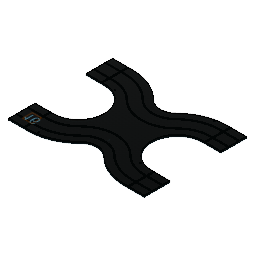
_10-16 (4-Way).ce05d46f-5f67-4321-aa04-e0567a5c2ecf (Autodesk Fusion 360 design; units mm, degrees)
Autodesk Fusion 360 part; units mm, degrees
note: some values were not read from the file. Set by a fixed rule: which sketch regions a step uses.
(part 1 of 2)
sketch "Sketch1" plane through (0, 0, 0) normal (0, 0, 1) x (1, 0, 0)
  line L0 (4241.8, -25.4) -> (3632.2, -25.4)
  line L1 (3632.2, -25.4) -> (3632.2, -838.2)
  line L2 (3632.2, -838.2) -> (4241.8, -838.2)
  line L3 (4241.8, -838.2) -> (4241.8, -25.4)
  line L4 (4241.8, -2438.4) -> (3632.2, -2438.4)
  line L5 (3632.2, -2438.4) -> (3632.2, -3251.2)
  line L6 (3632.2, -3251.2) -> (4241.8, -3251.2)
  line L7 (4241.8, -3251.2) -> (4241.8, -2438.4)
  line L8 (3632.2, -2438.4) -> (3632.2, -1638.3)
  line L9 (3632.2, -1638.3) -> (2870.2, -1638.3)
  circle A0 centre (3671.2525, -1638.3) radius 801.0525
  circle A1 centre (3632.2, -1638.3) radius 1612.9
  line L10 (0, 0) -> (609.6, 0)
  line L11 (609.6, 0) -> (609.6, -838.2)
  line L12 (609.6, -838.2) -> (0, -838.2)
  line L13 (0, -838.2) -> (0, 0)
  line L14 (0, -838.2) -> (0, -2438.4)
  line L15 (0, -2438.4) -> (609.6, -2438.4)
  line L16 (609.6, -2438.4) -> (609.6, -3276.6)
  line L17 (609.6, -3276.6) -> (0, -3276.6)
  line L18 (0, -3276.6) -> (0, -2438.4)
  line L19 (609.6, -838.2) -> (609.6, -2438.4)
  line L20 (609.6, -2438.4) -> (609.6, -1638.3)
  line L21 (609.6, -1638.3) -> (1371.6, -1638.3)
  circle A2 centre (570.5475, -1638.3) radius 801.0525
  circle A3 centre (609.6, -1638.3) radius 1638.3
  line L22 (3671.2525, -1638.3) -> (2870.2, -1638.3)
  line L23 (1371.6, -1638.3) -> (2870.2, -1638.3)
  line L24 (2120.9, -1638.3) -> (2120.9, -2635.25)
  line L25 (0, 0) -> (3390.4282, 0)
  line L26 (2065.6971, 0) -> (2065.6971, -635)
  circle A4 centre (2138.8294, -132.2917) radius 508
  circle A5 centre (2138.8294, -3144.3083) radius 508
  point P0 (2134.5605, -1039.5326)
  dimension "d8" = 609.6
  dimension "d9" = 812.8
  dimension "d12" = 812.8
  dimension "d13" = 800.1
  dimension "d14" = 762
  dimension "d15" = 609.6
  dimension "d16" = 838.2
  dimension "d17" = 1600.2
  dimension "d18" = 609.6
  dimension "d19" = 838.2
  dimension "d20" = 762
  dimension "d23" = 996.95
  dimension "d25" = 635
  dimension "d26" = 1016
  constraint horizontal L0
  constraint vertical L1
  constraint horizontal L2
  constraint vertical L3
  constraint horizontal L4
  constraint vertical L5
  constraint horizontal L6
  constraint vertical L7
  constraint perpendicular L2 L8
  constraint perpendicular L8 L9
  constraint coincident L1.end A0
  constraint coincident L9.end A0
  constraint coincident L4.end A0
  constraint coincident L5.end A1
  constraint tangent L6 A1
  constraint coincident L0.end A1
  constraint horizontal L10
  constraint vertical L11
  constraint horizontal L12
  constraint vertical L13
  constraint coincident L10.start L13.end
  constraint perpendicular L12 L14
  constraint horizontal L15
  constraint vertical L16
  constraint horizontal L17
  constraint vertical L18
  constraint midpoint L19 L20.end
  constraint perpendicular L19 L21
  constraint coincident L11.end A2
  constraint coincident L21.end A2
  constraint coincident L15.end A2
  constraint coincident L10.end A3
  constraint tangent L10 A3
  constraint coincident L16.end A3
  constraint coincident A0.centre L22.start
  constraint perpendicular L8 L22
  constraint parallel L22 L23
  constraint midpoint L23 L24.start
  constraint perpendicular L23 L24
  constraint coincident A3 P0
  constraint coincident A1 P0
  constraint perpendicular L3 L25
  constraint coincident L25 L26.start
  constraint perpendicular L25 L26
  constraint coincident L26.end A4
  constraint tangent A1 A4
  constraint tangent A3 A4
  constraint symmetric L23 A4 A5
  measures "d8" distance of L0.start L0.end
  measures "d9" distance of L0.start L2.end
  measures "d12" distance of L4.start L6.end
  measures "d13" distance of L4.end L8.end
  measures "d14" distance of L8.end L9.end
  measures "d15" distance of L10.start L10.end
  measures "d16" distance of L10.start L12.end
  measures "d17" distance of L12.end L14.end
  measures "d18" distance of L14.end L15.end
  measures "d19" distance of L14.end L17.end
  measures "d20" distance of L20.end L21.end
  measures "d23" distance of L24.start L24.end
  measures "d25" distance of L26.start L26.end
  measures "d26" diameter of A4
extrude "Extrude1" add sketch "Sketch1" along normal blind 50.8 contours L0 L3 A1 | L1 L2 L3 A0 A1 | L1 A0 A1 A3 L23 | A1 A3 A4 | L5 A0 A1 A3 L23 | A1 A3 L23 | A1 L11 A2 A3 L23 | L4 L5 L7 A0 A1 | L6 L7 A1 | A1 A3 L23 L24 | A1 L23 L24 | A1 L16 A2 A3 L23 L24 | A1 A3 A5 | L10 L13 A3 L25 | L11 L12 L13 A2 A3 | L15 L16 L18 A2 A3 | L17 L18 A3
sketch "Sketch2" plane through (0, 0, 0) normal (0, 0, -1) x (1, 0, 0)
  line L0 (2120.9, 2201.6993) -> (2120.9, 2270.7549)
  arc A0 (2134.5605, 2237.0674) -> (2120.9, 2270.7549) centre (609.6, 1638.3) ccw
  arc A1 (2134.5605, 2237.0674) -> (2120.9, 2201.6993) centre (3632.2, 1638.3) ccw
  line L1 (609.6, 3276.6) -> (0, 3276.6)
  line L2 (0, 3276.6) -> (0, 2438.4)
  line L3 (0, 2438.4) -> (531.495, 2438.4)
  arc A2 (531.495, 838.2) -> (531.495, 2438.4) centre (570.5475, 1638.3) ccw
  line L4 (531.495, 838.2) -> (0, 838.2)
  line L5 (0, 838.2) -> (0, 0)
  line L6 (0, 0) -> (609.6, 0)
  arc A3 (609.6, 0) -> (1776.8816, 488.7433) centre (609.6, 1638.3) ccw
  arc A4 (2496.523, 493.0122) -> (1776.8816, 488.7433) centre (2138.8294, 132.2917) ccw
  arc A5 (2496.523, 493.0122) -> (3632.2, 25.4) centre (3632.2, 1638.3) ccw
  line L7 (3632.2, 25.4) -> (4241.8, 25.4)
  line L8 (4241.8, 25.4) -> (4241.8, 838.2)
  line L9 (4241.8, 838.2) -> (3710.305, 838.2)
  arc A6 (3710.305, 2438.4) -> (3710.305, 838.2) centre (3671.2525, 1638.3) ccw
  line L10 (3710.305, 2438.4) -> (4241.8, 2438.4)
  line L11 (4241.8, 2438.4) -> (4241.8, 3251.2)
  line L12 (4241.8, 3251.2) -> (3632.2, 3251.2)
  arc A7 (3632.2, 3251.2) -> (2496.523, 2783.5878) centre (3632.2, 1638.3) ccw
  arc A8 (1776.8816, 2787.8567) -> (2496.523, 2783.5878) centre (2138.8294, 3144.3083) ccw
  arc A9 (1776.8816, 2787.8567) -> (609.6, 3276.6) centre (609.6, 1638.3) ccw
  line L13 (171.9803, 2701.7796) -> (461.5303, 2701.7796) construction
  line L14 (461.5303, 2701.7796) -> (461.5303, 3002.9116) construction
  line L15 (461.5303, 3002.9116) -> (171.9803, 3002.9116) construction
  line L16 (171.9803, 3002.9116) -> (171.9803, 2701.7796) construction
  dimension "d29" = 254
sketch "Sketch3" plane through (0, 0, 50.8) normal (0, 0, 1) x (-1, 0, 0)
  line L0 (-2120.9, 2270.7549) -> (-2120.9, 2201.6993)
  arc A0 (-2120.9, 2201.6993) -> (-2134.5605, 2237.0674) centre (-3632.2, 1638.3) ccw
  arc A1 (-2120.9, 2270.7549) -> (-2134.5605, 2237.0674) centre (-609.6, 1638.3) ccw
  line L1 (0, 3276.6) -> (-609.6, 3276.6)
  arc A2 (-609.6, 3276.6) -> (-1776.8816, 2787.8567) centre (-609.6, 1638.3) ccw
  arc A3 (-2496.523, 2783.5878) -> (-1776.8816, 2787.8567) centre (-2138.8294, 3144.3083) ccw
  arc A4 (-2496.523, 2783.5878) -> (-3632.2, 3251.2) centre (-3632.2, 1638.3) ccw
  line L2 (-3632.2, 3251.2) -> (-4241.8, 3251.2)
  line L3 (-4241.8, 3251.2) -> (-4241.8, 2438.4)
  line L4 (-4241.8, 2438.4) -> (-3710.305, 2438.4)
  arc A5 (-3710.305, 838.2) -> (-3710.305, 2438.4) centre (-3671.2525, 1638.3) ccw
  line L5 (-3710.305, 838.2) -> (-4241.8, 838.2)
  line L6 (-4241.8, 838.2) -> (-4241.8, 25.4)
  line L7 (-4241.8, 25.4) -> (-3632.2, 25.4)
  arc A6 (-3632.2, 25.4) -> (-2496.523, 493.0122) centre (-3632.2, 1638.3) ccw
  arc A7 (-1776.8816, 488.7433) -> (-2496.523, 493.0122) centre (-2138.8294, 132.2917) ccw
  arc A8 (-1776.8816, 488.7433) -> (-609.6, 0) centre (-609.6, 1638.3) ccw
  line L8 (-609.6, 0) -> (0, 0)
  line L9 (0, 0) -> (0, 838.2)
  line L10 (0, 838.2) -> (-531.495, 838.2)
  arc A9 (-531.495, 2438.4) -> (-531.495, 838.2) centre (-570.5475, 1638.3) ccw
  line L11 (-531.495, 2438.4) -> (0, 2438.4)
  line L12 (0, 2438.4) -> (0, 3276.6)
extrude "Extrude2" add sketch "Sketch3" against normal blind 50.8 contours L0 A0 A1
sketch "Sketch4" plane through (0, 0, 50.8) normal (0, 0, 1) x (-1, 0, 0)
  line L0 (0, 3276.6) -> (-609.6, 3276.6)
  arc A0 (-609.6, 3276.6) -> (-1776.8816, 2787.8567) centre (-609.6, 1638.3) ccw
  arc A1 (-2496.523, 2783.5878) -> (-1776.8816, 2787.8567) centre (-2138.8294, 3144.3083) ccw
  arc A2 (-2496.523, 2783.5878) -> (-3632.2, 3251.2) centre (-3632.2, 1638.3) ccw
  line L1 (-3632.2, 3251.2) -> (-4241.8, 3251.2)
  line L2 (-4241.8, 3251.2) -> (-4241.8, 2438.4)
  line L3 (-4241.8, 2438.4) -> (-3710.305, 2438.4)
  arc A3 (-3710.305, 838.2) -> (-3710.305, 2438.4) centre (-3671.2525, 1638.3) ccw
  line L4 (-3710.305, 838.2) -> (-4241.8, 838.2)
  line L5 (-4241.8, 838.2) -> (-4241.8, 25.4)
  line L6 (-4241.8, 25.4) -> (-3632.2, 25.4)
  arc A4 (-3632.2, 25.4) -> (-2496.523, 493.0122) centre (-3632.2, 1638.3) ccw
  arc A5 (-1776.8816, 488.7433) -> (-2496.523, 493.0122) centre (-2138.8294, 132.2917) ccw
  arc A6 (-1776.8816, 488.7433) -> (-609.6, 0) centre (-609.6, 1638.3) ccw
  line L7 (-609.6, 0) -> (0, 0)
  line L8 (0, 0) -> (0, 838.2)
  line L9 (0, 838.2) -> (-531.495, 838.2)
  arc A7 (-531.495, 2438.4) -> (-531.495, 838.2) centre (-570.5475, 1638.3) ccw
  line L10 (-531.495, 2438.4) -> (0, 2438.4)
  line L11 (0, 2438.4) -> (0, 3276.6)
  line L12 (-4241.8, 838.2) -> (-2590.8, 838.2)
  line L13 (-2590.8, 838.2) -> (-2590.8, 508)
  circle A8 centre (-2590.8, 508) radius 16
  dimension "d35" = 1651
  dimension "d37" = 330.2
  dimension "d38" = 32
  constraint coincident L4.end L5.start
  constraint perpendicular L5 L12
  constraint perpendicular L12 L13
  constraint coincident L13.end A8.centre
  measures "d35" distance of L4.end L12.end
  measures "d37" distance of L12.end L13.end
  measures "d38" diameter of A8
extrude "Extrude3" add sketch "Sketch4" along normal blind 0.0254 contours A8
sketch "Sketch5" plane through (0, 0, 50.8) normal (0, 0, 1) x (-1, 0, 0)
  circle A0 centre (-2590.8, 508) radius 16
  line L0 (0, 3276.6) -> (-609.6, 3276.6)
  arc A1 (-609.6, 3276.6) -> (-1776.8816, 2787.8567) centre (-609.6, 1638.3) ccw
  arc A2 (-2496.523, 2783.5878) -> (-1776.8816, 2787.8567) centre (-2138.8294, 3144.3083) ccw
  arc A3 (-2496.523, 2783.5878) -> (-3632.2, 3251.2) centre (-3632.2, 1638.3) ccw
  line L1 (-3632.2, 3251.2) -> (-4241.8, 3251.2)
  line L2 (-4241.8, 3251.2) -> (-4241.8, 2438.4)
  line L3 (-4241.8, 2438.4) -> (-3710.305, 2438.4)
  line L4 (-3710.305, 838.2) -> (-4241.8, 838.2)
  line L5 (-4241.8, 838.2) -> (-4241.8, 25.4)
  line L6 (-4241.8, 25.4) -> (-3632.2, 25.4)
  arc A4 (-1776.8816, 488.7433) -> (-2496.523, 493.0122) centre (-2138.8294, 132.2917) ccw
  arc A5 (-1776.8816, 488.7433) -> (-609.6, 0) centre (-609.6, 1638.3) ccw
  line L7 (-609.6, 0) -> (0, 0)
  line L8 (0, 0) -> (0, 838.2)
  line L9 (0, 838.2) -> (-531.495, 838.2)
  arc A6 (-531.495, 2438.4) -> (-531.495, 838.2) centre (-570.5475, 1638.3) ccw
  line L10 (-531.495, 2438.4) -> (0, 2438.4)
  line L11 (0, 2438.4) -> (0, 3276.6)
  line L12 (-3008.1535, 617.6738) -> (-2791.2306, 262.1613)
  line L13 (-3008.1535, 617.6738) -> (-2791.2306, 262.1613)
  line L14 (-2791.2306, 262.1613) -> (-2802.0718, 255.5463)
  line L15 (-2802.0718, 255.5463) -> (-3018.9947, 611.0588)
  line L16 (-3018.9947, 611.0588) -> (-3008.1535, 617.6738)
  point P0 (-3225.0764, 973.1864)
  point P1 (-2791.2306, 262.1613)
  point P2 (-3008.1535, 617.6738)
  dimension "d45" = 12.7
  constraint coincident P2 L12.start
  constraint coincident P1 L12.end
  constraint perpendicular L13 L14
  constraint parallel L13 L15
  constraint parallel L14 L16
  constraint parallel L12 L13
  measures "d45" distance of P2 L15.end
extrude "Extrude4" add sketch "Sketch5" along normal blind 0.0254 contours L12 L13 L14 L15 L16
extrude "Extrude5" cut sketch "Sketch5" along normal blind 0.0254 contours L12 L13 L14 L15 L16
extrude "Extrude6" add sketch "Sketch5" along normal blind 0.0254 contours L12 L13 L14 L15 L16
sketch "Sketch6" plane through (0, 0, 50.8) normal (0, 0, 1) x (-1, 0, 0)
  line L0 (-3018.9947, 611.0588) -> (-3008.1535, 617.6738)
  line L1 (-3008.1535, 617.6738) -> (-2791.2306, 262.1613)
  line L2 (-2791.2306, 262.1613) -> (-2802.0718, 255.5463)
  line L3 (-2802.0718, 255.5463) -> (-3018.9947, 611.0588)
  circle A0 centre (-2590.8, 508) radius 16
  line L4 (0, 3276.6) -> (-609.6, 3276.6)
  arc A1 (-609.6, 3276.6) -> (-1776.8816, 2787.8567) centre (-609.6, 1638.3) ccw
  arc A2 (-2496.523, 2783.5878) -> (-1776.8816, 2787.8567) centre (-2138.8294, 3144.3083) ccw
  arc A3 (-2496.523, 2783.5878) -> (-3632.2, 3251.2) centre (-3632.2, 1638.3) ccw
  line L5 (-3632.2, 3251.2) -> (-4241.8, 3251.2)
  line L6 (-4241.8, 3251.2) -> (-4241.8, 2438.4)
  line L7 (-4241.8, 2438.4) -> (-3710.305, 2438.4)
  arc A4 (-3710.305, 838.2) -> (-3710.305, 2438.4) centre (-3671.2525, 1638.3) ccw
  line L8 (-3710.305, 838.2) -> (-4241.8, 838.2)
  line L9 (-4241.8, 838.2) -> (-4241.8, 25.4)
  line L10 (-4241.8, 25.4) -> (-3632.2, 25.4)
  arc A5 (-3632.2, 25.4) -> (-2496.523, 493.0122) centre (-3632.2, 1638.3) ccw
  arc A6 (-1776.8816, 488.7433) -> (-2496.523, 493.0122) centre (-2138.8294, 132.2917) ccw
  arc A7 (-1776.8816, 488.7433) -> (-609.6, 0) centre (-609.6, 1638.3) ccw
  line L11 (-609.6, 0) -> (0, 0)
  line L12 (0, 0) -> (0, 838.2)
  line L13 (0, 838.2) -> (-531.495, 838.2)
  arc A8 (-531.495, 2438.4) -> (-531.495, 838.2) centre (-570.5475, 1638.3) ccw
  line L14 (-531.495, 2438.4) -> (0, 2438.4)
  line L15 (0, 2438.4) -> (0, 3276.6)
extrude "Extrude7" cut 1 faces at (2867.152, -378.4604, 50.8254) along direction (0, 0, -1) blind 0.0254
extrude "Extrude8" cut 1 faces at (2591.9868, -520.4548, 50.8254) along direction (0, 0, -1) blind 0.0254
sketch "Sketch7" plane through (0, 0, 50.8) normal (0, 0, 1) x (-1, 0, 0)
  line L0 (0, 3276.6) -> (-609.6, 3276.6)
  arc A0 (-609.6, 3276.6) -> (-1776.8816, 2787.8567) centre (-609.6, 1638.3) ccw
  arc A1 (-2496.523, 2783.5878) -> (-1776.8816, 2787.8567) centre (-2138.8294, 3144.3083) ccw
  arc A2 (-2496.523, 2783.5878) -> (-3632.2, 3251.2) centre (-3632.2, 1638.3) ccw
  line L1 (-3632.2, 3251.2) -> (-4241.8, 3251.2)
  line L2 (-4241.8, 3251.2) -> (-4241.8, 2438.4)
  line L3 (-4241.8, 2438.4) -> (-3710.305, 2438.4)
  arc A3 (-3710.305, 838.2) -> (-3710.305, 2438.4) centre (-3671.2525, 1638.3) ccw
  line L4 (-3710.305, 838.2) -> (-4241.8, 838.2)
  line L5 (-4241.8, 838.2) -> (-4241.8, 25.4)
  line L6 (-4241.8, 25.4) -> (-3632.2, 25.4)
  arc A4 (-3632.2, 25.4) -> (-2496.523, 493.0122) centre (-3632.2, 1638.3) ccw
  arc A5 (-1776.8816, 488.7433) -> (-2496.523, 493.0122) centre (-2138.8294, 132.2917) ccw
  arc A6 (-1776.8816, 488.7433) -> (-609.6, 0) centre (-609.6, 1638.3) ccw
  line L7 (-609.6, 0) -> (0, 0)
  line L8 (0, 0) -> (0, 838.2)
  line L9 (0, 838.2) -> (-531.495, 838.2)
  arc A7 (-531.495, 2438.4) -> (-531.495, 838.2) centre (-570.5475, 1638.3) ccw
  line L10 (-531.495, 2438.4) -> (0, 2438.4)
  line L11 (0, 2438.4) -> (0, 3276.6)
  line L12 (-3759.2, 741.3544) -> (-3759.2, 838.2)
  line L13 (-3759.2, 741.3544) -> (-3759.2, 25.4)
  line L14 (-3759.2, 838.2) -> (-3730.625, 838.2)
  line L15 (-3730.625, 838.2) -> (-3730.625, 25.4)
  line L16 (-3730.625, 25.4) -> (-3759.2, 25.4)
  line L17 (-3759.2, 838.2) -> (-3730.625, 838.2)
  line L18 (-3759.2, 838.2) -> (-3730.625, 838.2)
  line L19 (-3730.625, 838.2) -> (-3730.625, 25.4)
  line L20 (-3730.625, 25.4) -> (-3759.2, 25.4)
  line L21 (-3759.2, 25.4) -> (-3759.2, 838.2)
  constraint coincident L4 L12.end
  constraint perpendicular L4 L12
  constraint coincident L6 L13.end
  constraint perpendicular L6 L13
  constraint coincident L6 L15.end
  constraint perpendicular L6 L15
  constraint perpendicular L15 L17
  constraint horizontal L18
  constraint vertical L19
  constraint horizontal L20
  constraint vertical L21
extrude "Extrude9" add sketch "Sketch7" along normal blind 0.0254 contours L4 L6 L12 L13 L14 L15 L16 L17 L18 L19 L20 L21
sketch "Sketch8" plane through (0, 0, 50.8) normal (0, 0, 1) x (-1, 0, 0)
  line L0 (-3730.625, 838.2) -> (-3730.625, 25.4)
  line L1 (-3730.625, 25.4) -> (-3632.2, 25.4)
  arc A0 (-3632.2, 25.4) -> (-2496.523, 493.0122) centre (-3632.2, 1638.3) ccw
  arc A1 (-1776.8816, 488.7433) -> (-2496.523, 493.0122) centre (-2138.8294, 132.2917) ccw
  arc A2 (-1776.8816, 488.7433) -> (-609.6, 0) centre (-609.6, 1638.3) ccw
  line L2 (-609.6, 0) -> (0, 0)
  line L3 (0, 0) -> (0, 838.2)
  line L4 (0, 838.2) -> (-531.495, 838.2)
  arc A3 (-531.495, 2438.4) -> (-531.495, 838.2) centre (-570.5475, 1638.3) ccw
  line L5 (-531.495, 2438.4) -> (0, 2438.4)
  line L6 (0, 2438.4) -> (0, 3276.6)
  line L7 (0, 3276.6) -> (-609.6, 3276.6)
  arc A4 (-609.6, 3276.6) -> (-1776.8816, 2787.8567) centre (-609.6, 1638.3) ccw
  arc A5 (-2496.523, 2783.5878) -> (-1776.8816, 2787.8567) centre (-2138.8294, 3144.3083) ccw
  arc A6 (-2496.523, 2783.5878) -> (-3632.2, 3251.2) centre (-3632.2, 1638.3) ccw
  line L8 (-3632.2, 3251.2) -> (-4241.8, 3251.2)
  line L9 (-4241.8, 3251.2) -> (-4241.8, 2438.4)
  line L10 (-4241.8, 2438.4) -> (-3710.305, 2438.4)
  arc A7 (-3710.305, 838.2) -> (-3710.305, 2438.4) centre (-3671.2525, 1638.3) ccw
  line L11 (-3710.305, 838.2) -> (-3730.625, 838.2)
sketch "Sketch9" plane through (0, 0, 50.8) normal (0, 0, 1) x (-1, 0, 0)
  line L0 (0, 431.8) -> (-482.6, 431.8)
  line L1 (-482.6, 431.8) -> (-482.6, 838.2)
  line L2 (-482.6, 838.2) -> (-511.175, 838.2)
  line L3 (-511.175, 838.2) -> (-511.175, -0.0124)
  line L4 (-511.175, -0.0124) -> (-482.6, -0.0124)
  line L5 (-482.6, -0.0124) -> (-482.6, 838.2)
  line L6 (0, 2870.2) -> (-482.6, 2870.2)
  line L7 (-4241.7999, 2844.8) -> (-3759.1999, 2844.8)
  line L8 (-3759.1999, 2844.8) -> (-3730.6249, 2844.8)
  line L9 (-3730.6249, 2844.8) -> (-3730.6249, 2438.5075)
  line L10 (-3730.6249, 2438.5075) -> (-3759.1999, 2438.5075)
  line L11 (-3759.1999, 2438.5075) -> (-3759.1999, 2844.8)
  line L12 (-3730.6249, 2844.8) -> (-3759.1999, 2844.8)
  line L13 (-3759.1999, 2844.8) -> (-3759.1999, 3251.2)
  line L14 (-3759.1999, 3251.2) -> (-3730.6249, 3251.2)
  line L15 (-3730.6249, 3251.2) -> (-3730.6249, 2844.8)
  line L16 (-482.6, 2870.2) -> (-511.175, 2870.2)
  line L17 (-511.175, 2870.2) -> (-511.175, 2438.6051)
  line L18 (-511.175, 2438.6051) -> (-482.6, 2438.6051)
  line L19 (-482.6, 2438.6051) -> (-482.6, 2870.2)
  line L20 (-482.6, 2870.2) -> (-511.175, 2870.2)
  line L21 (-511.175, 2870.2) -> (-511.175, 3276.173)
  line L22 (-511.175, 3276.173) -> (-482.6, 3276.173)
  line L23 (-482.6, 3276.173) -> (-482.6, 2870.2)
  line L24 (-3730.625, 838.2) -> (-3730.625, 25.4)
  line L25 (-3730.625, 25.4) -> (-3632.2, 25.4)
  arc A0 (-3632.2, 25.4) -> (-2496.523, 493.0122) centre (-3632.2, 1638.3) ccw
  arc A1 (-1776.8816, 488.7433) -> (-2496.523, 493.0122) centre (-2138.8294, 132.2917) ccw
  arc A2 (-1776.8816, 488.7433) -> (-609.6, 0) centre (-609.6, 1638.3) ccw
  line L26 (-609.6, 0) -> (0, 0)
  line L27 (0, 0) -> (0, 838.2)
  line L28 (0, 838.2) -> (-531.495, 838.2)
  arc A3 (-531.495, 2438.4) -> (-531.495, 838.2) centre (-570.5475, 1638.3) ccw
  line L29 (-531.495, 2438.4) -> (0, 2438.4)
  line L30 (0, 2438.4) -> (0, 3276.6)
  line L31 (0, 3276.6) -> (-609.6, 3276.6)
  arc A4 (-609.6, 3276.6) -> (-1776.8816, 2787.8567) centre (-609.6, 1638.3) ccw
  arc A5 (-2496.523, 2783.5878) -> (-1776.8816, 2787.8567) centre (-2138.8294, 3144.3083) ccw
  arc A6 (-2496.523, 2783.5878) -> (-3632.2, 3251.2) centre (-3632.2, 1638.3) ccw
  line L32 (-3632.2, 3251.2) -> (-4241.8, 3251.2)
  line L33 (-4241.8, 3251.2) -> (-4241.8, 2438.4)
  line L34 (-4241.8, 2438.4) -> (-3710.305, 2438.4)
  arc A7 (-3710.305, 838.2) -> (-3710.305, 2438.4) centre (-3671.2525, 1638.3) ccw
  line L35 (-3710.305, 838.2) -> (-3730.625, 838.2)
  line L36 (-4241.8, 25.4) -> (-3632.2, 25.4)
  line L37 (-3710.305, 838.2) -> (-4241.8, 838.2)
  line L38 (-4241.8, 838.2) -> (-4241.8, 25.4)
  line L39 (-63.5, 774.7) -> (-529.9758, 774.7)
  arc A8 (-529.9758, 2501.9) -> (-529.9758, 774.7) centre (-570.5475, 1638.3) ccw
  line L40 (-529.9758, 2501.9) -> (-63.5, 2501.9)
  line L41 (-63.5, 2501.9) -> (-63.5, 3213.1)
  line L42 (-63.5, 3213.1) -> (-609.6, 3213.1)
  arc A9 (-609.6, 3213.1) -> (-1731.6381, 2743.3002) centre (-609.6, 1638.3) ccw
  arc A10 (-2541.2347, 2738.4977) -> (-1731.6381, 2743.3002) centre (-2138.8294, 3144.3083) ccw
  arc A11 (-2541.2347, 2738.4977) -> (-3632.2, 3187.7) centre (-3632.2, 1638.3) ccw
  line L43 (-3632.2, 3187.7) -> (-4178.3, 3187.7)
  line L44 (-4178.3, 3187.7) -> (-4178.3, 2501.9)
  line L45 (-4178.3, 2501.9) -> (-3711.8242, 2501.9)
  arc A12 (-3667.125, 773.7574) -> (-3711.8242, 2501.9) centre (-3671.2525, 1638.3) ccw
  line L46 (-3667.125, 773.7574) -> (-3667.125, 88.9)
  line L47 (-3667.125, 88.9) -> (-3632.2, 88.9)
  arc A13 (-3632.2, 88.9) -> (-2541.2347, 538.1023) centre (-3632.2, 1638.3) ccw
  arc A14 (-1731.6381, 533.2998) -> (-2541.2347, 538.1023) centre (-2138.8294, 132.2917) ccw
  arc A15 (-1731.6381, 533.2998) -> (-609.6, 63.5) centre (-609.6, 1638.3) ccw
  line L48 (-609.6, 63.5) -> (-63.5, 63.5)
  line L49 (-63.5, 63.5) -> (-63.5, 774.7)
  circle A16 centre (-3302, 2420.0312) radius 16
  circle A17 centre (-863.6, 3192.4811) radius 16
  circle A18 centre (-914.4, 845.0683) radius 16
  circle A19 centre (-3314.7, 121.7796) radius 16
  dimension "d60" = 482.6
  dimension "d61" = 28.575
  dimension "d62" = 482.6
  dimension "d63" = 482.6
  dimension "d64" = 28.575
  dimension "d65" = 28.575
  dimension "d66" = 63.5
  dimension "d70" = 32
  dimension "d72" = 32
  dimension "d74" = 32
  dimension "d76" = 32
  constraint horizontal L0
  constraint perpendicular L0 L1
  constraint horizontal L2
  constraint vertical L3
  constraint horizontal L4
  constraint vertical L5
  constraint horizontal L6
  constraint horizontal L7
  constraint horizontal L8
  constraint vertical L9
  constraint horizontal L10
  constraint vertical L11
  constraint horizontal L12
  constraint vertical L13
  constraint horizontal L14
  constraint vertical L15
  constraint horizontal L16
  constraint vertical L17
  constraint horizontal L18
  constraint vertical L19
  constraint horizontal L20
  constraint vertical L21
  constraint horizontal L22
  constraint vertical L23
  measures "d60" distance of L0.start L0.end
  measures "d61" distance of L1.end L2.end
  measures "d62" distance of L6.start L6.end
  measures "d63" distance of L7.start L7.end
  measures "d64" distance of L7.end L8.end
  measures "d65" distance of L6.end L16.end
  measures "d70" diameter of A16
  measures "d72" diameter of A17
  measures "d74" diameter of A18
  measures "d76" diameter of A19
extrude "Extrude10" add sketch "Sketch9" along normal blind 0.0254 contours L1 L3 L5 L39 L48 | L3 L5 L26 L48 | L1 L2 L3 L5 L28 L39 | L17 L18 L19 L40 | L16 L17 L19 L20 L40 | L16 L20 L21 L23 L42 | L21 L22 L23 L42 | L13 L14 L15 L32 L43 | L8 L12 L13 L15 L43 | L8 L9 L11 L12 L45 | L9 L10 L11 L45
extrude "Extrude11" add sketch "Sketch9" along normal blind 0.0254 contours A8 A18 | A8 A18 | A13 A19 | A13 A19 | A9 A17 | A9 A17 | A12 A16 | A12 A16
sketch "Sketch10" plane through (0, 0, 50.8) normal (0, 0, 1) x (-1, 0, 0)
  circle A0 centre (-3314.7, 121.7796) radius 16
  circle A1 centre (-3302, 2420.0312) radius 16
  circle A2 centre (-914.4, 845.0683) radius 16
  circle A3 centre (-863.6, 3192.4811) radius 16
  line L0 (-482.6, 838.2) -> (-482.6, 0)
  line L1 (-482.6, 0) -> (0, 0)
  line L2 (0, 0) -> (0, 838.2)
  line L3 (0, 838.2) -> (-531.495, 838.2)
  arc A4 (-531.495, 2438.4) -> (-531.495, 838.2) centre (-570.5475, 1638.3) ccw
  line L4 (-531.495, 2438.4) -> (0, 2438.4)
  line L5 (0, 2438.4) -> (0, 3276.6)
  line L6 (0, 3276.6) -> (-609.6, 3276.6)
  arc A5 (-609.6, 3276.6) -> (-1776.8816, 2787.8567) centre (-609.6, 1638.3) ccw
  arc A6 (-2496.523, 2783.5878) -> (-1776.8816, 2787.8567) centre (-2138.8294, 3144.3083) ccw
  arc A7 (-2496.523, 2783.5878) -> (-3632.2, 3251.2) centre (-3632.2, 1638.3) ccw
  line L7 (-3632.2, 3251.2) -> (-4241.8, 3251.2)
  line L8 (-4241.8, 3251.2) -> (-4241.8, 2438.4)
  line L9 (-4241.8, 2438.4) -> (-3710.305, 2438.4)
  arc A8 (-3710.305, 838.2) -> (-3710.305, 2438.4) centre (-3671.2525, 1638.3) ccw
  line L10 (-3710.305, 838.2) -> (-3730.625, 838.2)
  line L11 (-3730.625, 838.2) -> (-3730.625, 25.4)
  line L12 (-3730.625, 25.4) -> (-3632.2, 25.4)
  arc A9 (-3632.2, 25.4) -> (-2496.523, 493.0122) centre (-3632.2, 1638.3) ccw
  arc A10 (-1776.8816, 488.7433) -> (-2496.523, 493.0122) centre (-2138.8294, 132.2917) ccw
  arc A11 (-1776.8816, 488.7433) -> (-609.6, 0) centre (-609.6, 1638.3) ccw
  line L13 (-609.6, 0) -> (-511.175, 0)
  line L14 (-511.175, 0) -> (-511.175, 838.2)
  line L15 (-511.175, 838.2) -> (-482.6, 838.2)
  line L16 (-511.175, 3276.173) -> (-482.6, 3276.173)
  line L17 (-482.6, 3276.173) -> (-482.6, 2438.6051)
  line L18 (-482.6, 2438.6051) -> (-511.175, 2438.6051)
  line L19 (-511.175, 2438.6051) -> (-511.175, 3276.173)
  line L20 (-3730.6249, 3251.2) -> (-3730.6249, 2438.5075)
  line L21 (-3730.6249, 2438.5075) -> (-3759.1999, 2438.5075)
  line L22 (-3759.1999, 2438.5075) -> (-3759.1999, 3251.2)
  line L23 (-3759.1999, 3251.2) -> (-3730.6249, 3251.2)
  arc A12 (-1611.7429, 651.3744) -> (-609.6, 231.775) centre (-609.6, 1638.3) ccw
  line L24 (-609.6, 231.775) -> (-511.175, 231.775)
  arc A13 (-1598.1699, 664.7414) -> (-609.6, 250.825) centre (-609.6, 1638.3) ccw
  line L25 (-609.6, 250.825) -> (-511.175, 250.825)
  arc A14 (-1598.1699, 664.7414) -> (-2673.1342, 671.118) centre (-2138.8294, 132.2917) ccw
  arc A15 (-1611.7429, 651.3744) -> (-2659.7206, 657.591) centre (-2138.8294, 132.2917) ccw
  arc A16 (-3632.2, 257.175) -> (-2659.7206, 657.591) centre (-3632.2, 1638.3) ccw
  line L26 (-3730.625, 257.175) -> (-3632.2, 257.175)
  line L27 (-3730.625, 276.225) -> (-3632.2, 276.225)
  arc A17 (-3632.2, 276.225) -> (-2673.1342, 671.118) centre (-3632.2, 1638.3) ccw
  dimension "d79" = -231.775
  dimension "d80" = -250.825
  dimension "d81" = 250.825
  dimension "d82" = 231.775
  dimension "d85" = -250.825
extrude "Extrude12" add sketch "Sketch10" along normal blind 0.0279 contours L11 L14 A12 L24 A13 L25 A14 A15 A16 L26 L27 A17
sketch "Sketch11" plane through (0, 0, 0) normal (0, 0, -1) x (1, 0, 0)
sketch "Sketch12" plane through (0, 0, 50.8) normal (0, 0, 1) x (-1, 0, 0)
  line L0 (-609.6, 250.825) -> (-511.175, 250.825)
  line L1 (-511.175, 250.825) -> (-511.175, 838.2)
  line L2 (-511.175, 838.2) -> (-482.6, 838.2)
  line L3 (-482.6, 838.2) -> (-482.6, 0)
  line L4 (-482.6, 0) -> (0, 0)
  line L5 (0, 0) -> (0, 838.2)
  line L6 (0, 838.2) -> (-531.495, 838.2)
  arc A0 (-531.495, 2438.4) -> (-531.495, 838.2) centre (-570.5475, 1638.3) ccw
  line L7 (-531.495, 2438.4) -> (0, 2438.4)
  line L8 (0, 2438.4) -> (0, 3276.6)
  line L9 (0, 3276.6) -> (-609.6, 3276.6)
  arc A1 (-609.6, 3276.6) -> (-1776.8816, 2787.8567) centre (-609.6, 1638.3) ccw
  arc A2 (-2496.523, 2783.5878) -> (-1776.8816, 2787.8567) centre (-2138.8294, 3144.3083) ccw
  arc A3 (-2496.523, 2783.5878) -> (-3632.2, 3251.2) centre (-3632.2, 1638.3) ccw
  line L10 (-3632.2, 3251.2) -> (-4241.8, 3251.2)
  line L11 (-4241.8, 3251.2) -> (-4241.8, 2438.4)
  line L12 (-4241.8, 2438.4) -> (-3710.305, 2438.4)
  arc A4 (-3710.305, 838.2) -> (-3710.305, 2438.4) centre (-3671.2525, 1638.3) ccw
  line L13 (-3710.305, 838.2) -> (-3730.625, 838.2)
  line L14 (-3730.625, 838.2) -> (-3730.625, 276.225)
  line L15 (-3730.625, 276.225) -> (-3632.2, 276.225)
  arc A5 (-3632.2, 276.225) -> (-2673.1342, 671.118) centre (-3632.2, 1638.3) ccw
  arc A6 (-1598.1699, 664.7414) -> (-2673.1342, 671.118) centre (-2138.8294, 132.2917) ccw
  arc A7 (-1598.1699, 664.7414) -> (-609.6, 250.825) centre (-609.6, 1638.3) ccw
  circle A8 centre (-3302, 2420.0312) radius 16
  circle A9 centre (-914.4, 845.0683) radius 16
  circle A10 centre (-863.6, 3192.4811) radius 16
  line L16 (-511.175, 3276.173) -> (-482.6, 3276.173)
  line L17 (-482.6, 3276.173) -> (-482.6, 2438.6051)
  line L18 (-482.6, 2438.6051) -> (-511.175, 2438.6051)
  line L19 (-511.175, 2438.6051) -> (-511.175, 3276.173)
  line L20 (-3730.6249, 3251.2) -> (-3730.6249, 2438.5075)
  line L21 (-3730.6249, 2438.5075) -> (-3759.1999, 2438.5075)
  line L22 (-3759.1999, 2438.5075) -> (-3759.1999, 3251.2)
  line L23 (-3759.1999, 3251.2) -> (-3730.6249, 3251.2)
  line L24 (-482.6, 250.825) -> (0, 250.825)
  line L25 (-482.6, 231.775) -> (0, 231.775)
  dimension "d89" = -231.775
extrude "Extrude13" add sketch "Sketch12" along normal blind 0.0279 contours L3 L5 L24 L25
sketch "Sketch13" plane through (0, 0, 50.8) normal (0, 0, 1) x (-1, 0, 0)
  line L0 (-482.6, 250.825) -> (0, 250.825)
  line L1 (0, 250.825) -> (0, 838.2)
  line L2 (0, 838.2) -> (-531.495, 838.2)
  arc A0 (-531.495, 2438.4) -> (-531.495, 838.2) centre (-570.5475, 1638.3) ccw
  line L3 (-531.495, 2438.4) -> (0, 2438.4)
  line L4 (0, 2438.4) -> (0, 3276.6)
  line L5 (0, 3276.6) -> (-609.6, 3276.6)
  arc A1 (-609.6, 3276.6) -> (-1776.8816, 2787.8567) centre (-609.6, 1638.3) ccw
  arc A2 (-2496.523, 2783.5878) -> (-1776.8816, 2787.8567) centre (-2138.8294, 3144.3083) ccw
  arc A3 (-2496.523, 2783.5878) -> (-3632.2, 3251.2) centre (-3632.2, 1638.3) ccw
  line L6 (-3632.2, 3251.2) -> (-4241.8, 3251.2)
  line L7 (-4241.8, 3251.2) -> (-4241.8, 2438.4)
  line L8 (-4241.8, 2438.4) -> (-3710.305, 2438.4)
  arc A4 (-3710.305, 838.2) -> (-3710.305, 2438.4) centre (-3671.2525, 1638.3) ccw
  line L9 (-3710.305, 838.2) -> (-3730.625, 838.2)
  line L10 (-3730.625, 838.2) -> (-3730.625, 276.225)
  line L11 (-3730.625, 276.225) -> (-3632.2, 276.225)
  arc A5 (-3632.2, 276.225) -> (-2673.1342, 671.118) centre (-3632.2, 1638.3) ccw
  arc A6 (-1598.1699, 664.7414) -> (-2673.1342, 671.118) centre (-2138.8294, 132.2917) ccw
  arc A7 (-1598.1699, 664.7414) -> (-609.6, 250.825) centre (-609.6, 1638.3) ccw
  line L12 (-609.6, 250.825) -> (-511.175, 250.825)
  line L13 (-511.175, 250.825) -> (-511.175, 838.2)
  line L14 (-511.175, 838.2) -> (-482.6, 838.2)
  line L15 (-482.6, 838.2) -> (-482.6, 250.825)
  circle A8 centre (-3302, 2420.0312) radius 16
  circle A9 centre (-914.4, 845.0683) radius 16
  circle A10 centre (-863.6, 3192.4811) radius 16
  line L16 (-511.175, 3276.173) -> (-482.6, 3276.173)
  line L17 (-482.6, 3276.173) -> (-482.6, 2438.6051)
  line L18 (-482.6, 2438.6051) -> (-511.175, 2438.6051)
  line L19 (-511.175, 2438.6051) -> (-511.175, 3276.173)
  line L20 (-3730.6249, 3251.2) -> (-3730.6249, 2438.5075)
  line L21 (-3730.6249, 2438.5075) -> (-3759.1999, 2438.5075)
  line L22 (-3759.1999, 2438.5075) -> (-3759.1999, 3251.2)
  line L23 (-3759.1999, 3251.2) -> (-3730.6249, 3251.2)
  line L24 (0, 587.375) -> (-531.495, 587.375)
  line L25 (0, 606.425) -> (-531.495, 606.425)
  dimension "d92" = -250.825
  dimension "d93" = -231.775
extrude "Extrude14" add sketch "Sketch13" along normal blind 0.0279 contours L1 L15 L24 L25
sketch "Sketch14" plane through (0, 0, 50.8) normal (0, 0, 1) x (-1, 0, 0)
  line L0 (-482.6, 606.425) -> (0, 606.425)
  line L1 (0, 606.425) -> (0, 838.2)
  line L2 (0, 838.2) -> (-531.495, 838.2)
  arc A0 (-531.495, 2438.4) -> (-531.495, 838.2) centre (-570.5475, 1638.3) ccw
  line L3 (-531.495, 2438.4) -> (0, 2438.4)
  line L4 (0, 2438.4) -> (0, 3276.6)
  line L5 (0, 3276.6) -> (-609.6, 3276.6)
  arc A1 (-609.6, 3276.6) -> (-1776.8816, 2787.8567) centre (-609.6, 1638.3) ccw
  arc A2 (-2496.523, 2783.5878) -> (-1776.8816, 2787.8567) centre (-2138.8294, 3144.3083) ccw
  arc A3 (-2496.523, 2783.5878) -> (-3632.2, 3251.2) centre (-3632.2, 1638.3) ccw
  line L6 (-3632.2, 3251.2) -> (-4241.8, 3251.2)
  line L7 (-4241.8, 3251.2) -> (-4241.8, 2438.4)
  line L8 (-4241.8, 2438.4) -> (-3710.305, 2438.4)
  arc A4 (-3710.305, 838.2) -> (-3710.305, 2438.4) centre (-3671.2525, 1638.3) ccw
  line L9 (-3710.305, 838.2) -> (-3730.625, 838.2)
  line L10 (-3730.625, 838.2) -> (-3730.625, 276.225)
  line L11 (-3730.625, 276.225) -> (-3632.2, 276.225)
  arc A5 (-3632.2, 276.225) -> (-2673.1342, 671.118) centre (-3632.2, 1638.3) ccw
  arc A6 (-1598.1699, 664.7414) -> (-2673.1342, 671.118) centre (-2138.8294, 132.2917) ccw
  arc A7 (-1598.1699, 664.7414) -> (-609.6, 250.825) centre (-609.6, 1638.3) ccw
  line L12 (-609.6, 250.825) -> (-511.175, 250.825)
  line L13 (-511.175, 250.825) -> (-511.175, 838.2)
  line L14 (-511.175, 838.2) -> (-482.6, 838.2)
  line L15 (-482.6, 838.2) -> (-482.6, 606.425)
  circle A8 centre (-3302, 2420.0312) radius 16
  circle A9 centre (-914.4, 845.0683) radius 16
  circle A10 centre (-863.6, 3192.4811) radius 16
  line L16 (-511.175, 3276.173) -> (-482.6, 3276.173)
  line L17 (-482.6, 3276.173) -> (-482.6, 2438.6051)
  line L18 (-482.6, 2438.6051) -> (-511.175, 2438.6051)
  line L19 (-511.175, 2438.6051) -> (-511.175, 3276.173)
  line L20 (-3730.6249, 3251.2) -> (-3730.6249, 2438.5075)
  line L21 (-3730.6249, 2438.5075) -> (-3759.1999, 2438.5075)
  line L22 (-3759.1999, 2438.5075) -> (-3759.1999, 3251.2)
  line L23 (-3759.1999, 3251.2) -> (-3730.6249, 3251.2)
  arc A11 (-1358.3795, 900.8906) -> (-609.6, 587.375) centre (-609.6, 1638.3) ccw
  line L24 (-609.6, 587.375) -> (-511.175, 587.375)
  arc A12 (-1358.3795, 900.8906) -> (-2910.1061, 910.0954) centre (-2138.8294, 132.2917) ccw
  line L25 (-3730.625, 612.775) -> (-3632.2, 612.775)
  arc A13 (-3632.2, 612.775) -> (-2910.1061, 910.0954) centre (-3632.2, 1638.3) ccw
  arc A14 (-1344.8064, 914.2575) -> (-609.6, 606.425) centre (-609.6, 1638.3) ccw
  line L26 (-609.6, 606.425) -> (-511.175, 606.425)
  arc A15 (-1344.8064, 914.2575) -> (-2923.5196, 923.6224) centre (-2138.8294, 132.2917) ccw
  line L27 (-3730.625, 631.825) -> (-3632.2, 631.825)
  arc A16 (-3632.2, 631.825) -> (-2923.5196, 923.6224) centre (-3632.2, 1638.3) ccw
  arc A17 (-3716.0065, 587.375) -> (-3722.5331, 2688.9268) centre (-3671.2525, 1638.3) ccw
  line L28 (-3716.0065, 587.375) -> (-3730.625, 587.375)
  arc A18 (-3715.5992, 606.425) -> (-3721.6044, 2669.8994) centre (-3671.2525, 1638.3) ccw
  line L29 (-3715.5992, 606.425) -> (-3730.625, 606.425)
  dimension "d96" = -336.55
  dimension "d97" = 336.55
  dimension "d98" = -336.55
  dimension "d99" = -355.6
  dimension "d100" = 355.6
  dimension "d101" = -355.6
  dimension "d138" = -250.825
  dimension "d139" = -231.775
sketch "Sketch15" plane through (0, 0, 50.8) normal (0, 0, 1) x (-1, 0, 0)
  line L0 (-511.175, 250.825) -> (-511.175, 838.2)
  line L1 (-511.175, 838.2) -> (-482.6, 838.2)
  line L2 (-482.6, 838.2) -> (-482.6, 606.425)
  line L3 (-482.6, 606.425) -> (0, 606.425)
  line L4 (0, 606.425) -> (0, 838.2)
  line L5 (0, 838.2) -> (-531.495, 838.2)
  arc A0 (-531.495, 2438.4) -> (-531.495, 838.2) centre (-570.5475, 1638.3) ccw
  line L6 (-531.495, 2438.4) -> (0, 2438.4)
  line L7 (0, 2438.4) -> (0, 3276.6)
  line L8 (0, 3276.6) -> (-609.6, 3276.6)
  arc A1 (-609.6, 3276.6) -> (-1776.8816, 2787.8567) centre (-609.6, 1638.3) ccw
  arc A2 (-2496.523, 2783.5878) -> (-1776.8816, 2787.8567) centre (-2138.8294, 3144.3083) ccw
  arc A3 (-2496.523, 2783.5878) -> (-3632.2, 3251.2) centre (-3632.2, 1638.3) ccw
  line L9 (-3632.2, 3251.2) -> (-4241.8, 3251.2)
  line L10 (-4241.8, 3251.2) -> (-4241.8, 2438.4)
  line L11 (-4241.8, 2438.4) -> (-3710.305, 2438.4)
  arc A4 (-3710.305, 838.2) -> (-3710.305, 2438.4) centre (-3671.2525, 1638.3) ccw
  line L12 (-3710.305, 838.2) -> (-3730.625, 838.2)
  line L13 (-3730.625, 838.2) -> (-3730.625, 276.225)
  circle A5 centre (-3302, 2420.0312) radius 16
  circle A6 centre (-914.4, 845.0683) radius 16
  circle A7 centre (-863.6, 3192.4811) radius 16
  line L14 (-511.175, 3276.173) -> (-482.6, 3276.173)
  line L15 (-482.6, 3276.173) -> (-482.6, 2438.6051)
  line L16 (-482.6, 2438.6051) -> (-511.175, 2438.6051)
  line L17 (-511.175, 2438.6051) -> (-511.175, 3276.173)
  line L18 (-3730.6249, 3251.2) -> (-3730.6249, 2438.5075)
  line L19 (-3730.6249, 2438.5075) -> (-3759.1999, 2438.5075)
  line L20 (-3759.1999, 2438.5075) -> (-3759.1999, 3251.2)
  line L21 (-3759.1999, 3251.2) -> (-3730.6249, 3251.2)
  line L22 (-531.495, 2689.225) -> (0, 2689.225)
  line L23 (-531.495, 2670.175) -> (0, 2670.175)
  line L24 (-3730.625, 276.225) -> (-3632.2, 276.225)
  arc A8 (-3632.2, 276.225) -> (-2673.1342, 671.118) centre (-3632.2, 1638.3) ccw
  arc A9 (-1598.1699, 664.7414) -> (-2673.1342, 671.118) centre (-2138.8294, 132.2917) ccw
  arc A10 (-1598.1699, 664.7414) -> (-609.6, 250.825) centre (-609.6, 1638.3) ccw
  line L25 (-609.6, 250.825) -> (-511.175, 250.825)
  dimension "d104" = -250.825
  dimension "d105" = -231.775
extrude "Extrude16" add sketch "Sketch15" along normal blind 0.0279 contours L7 L15 L22 L23
sketch "Sketch16" plane through (0, 0, 50.8) normal (0, 0, 1) x (-1, 0, 0)
  line L0 (-482.6, 2689.225) -> (0, 2689.225)
  line L1 (0, 2689.225) -> (0, 3276.6)
  line L2 (0, 3276.6) -> (-609.6, 3276.6)
  arc A0 (-609.6, 3276.6) -> (-1776.8816, 2787.8567) centre (-609.6, 1638.3) ccw
  arc A1 (-2496.523, 2783.5878) -> (-1776.8816, 2787.8567) centre (-2138.8294, 3144.3083) ccw
  arc A2 (-2496.523, 2783.5878) -> (-3632.2, 3251.2) centre (-3632.2, 1638.3) ccw
  line L3 (-3632.2, 3251.2) -> (-4241.8, 3251.2)
  line L4 (-4241.8, 3251.2) -> (-4241.8, 2438.4)
  line L5 (-4241.8, 2438.4) -> (-3710.305, 2438.4)
  arc A3 (-3710.305, 838.2) -> (-3710.305, 2438.4) centre (-3671.2525, 1638.3) ccw
  line L6 (-3710.305, 838.2) -> (-3730.625, 838.2)
  line L7 (-3730.625, 838.2) -> (-3730.625, 276.225)
  line L8 (-511.175, 250.825) -> (-511.175, 838.2)
  line L9 (-511.175, 838.2) -> (-482.6, 838.2)
  line L10 (-482.6, 838.2) -> (-482.6, 606.425)
  line L11 (-482.6, 606.425) -> (0, 606.425)
  line L12 (0, 606.425) -> (0, 838.2)
  line L13 (0, 838.2) -> (-531.495, 838.2)
  arc A4 (-531.495, 2438.4) -> (-531.495, 838.2) centre (-570.5475, 1638.3) ccw
  line L14 (-531.495, 2438.4) -> (0, 2438.4)
  line L15 (0, 2438.4) -> (0, 2670.175)
  line L16 (0, 2670.175) -> (-482.6, 2670.175)
  line L17 (-482.6, 2670.175) -> (-482.6, 2438.6051)
  line L18 (-482.6, 2438.6051) -> (-511.175, 2438.6051)
  line L19 (-511.175, 2438.6051) -> (-511.175, 3276.173)
  line L20 (-511.175, 3276.173) -> (-482.6, 3276.173)
  line L21 (-482.6, 3276.173) -> (-482.6, 2689.225)
  circle A5 centre (-3302, 2420.0312) radius 16
  circle A6 centre (-914.4, 845.0683) radius 16
  circle A7 centre (-863.6, 3192.4811) radius 16
  line L22 (-3730.6249, 3251.2) -> (-3730.6249, 2438.5075)
  line L23 (-3730.6249, 2438.5075) -> (-3759.1999, 2438.5075)
  line L24 (-3759.1999, 2438.5075) -> (-3759.1999, 3251.2)
  line L25 (-3759.1999, 3251.2) -> (-3730.6249, 3251.2)
  line L26 (0, 3025.775) -> (-609.6, 3025.775)
  line L27 (0, 3044.825) -> (-609.6, 3044.825)
  line L28 (-3730.625, 276.225) -> (-3632.2, 276.225)
  arc A8 (-3632.2, 276.225) -> (-2673.1342, 671.118) centre (-3632.2, 1638.3) ccw
  arc A9 (-1598.1699, 664.7414) -> (-2673.1342, 671.118) centre (-2138.8294, 132.2917) ccw
  arc A10 (-1598.1699, 664.7414) -> (-609.6, 250.825) centre (-609.6, 1638.3) ccw
  line L29 (-609.6, 250.825) -> (-511.175, 250.825)
  dimension "d108" = -250.825
  dimension "d109" = -231.775
extrude "Extrude17" add sketch "Sketch16" along normal blind 0.0279 contours L1 L21 L26 L27
sketch "Sketch17" plane through (0, 0, 50.8) normal (0, 0, 1) x (-1, 0, 0)
  line L0 (-482.6, 3044.825) -> (0, 3044.825)
  line L1 (0, 3044.825) -> (0, 3276.6)
  line L2 (0, 3276.6) -> (-609.6, 3276.6)
  arc A0 (-609.6, 3276.6) -> (-1776.8816, 2787.8567) centre (-609.6, 1638.3) ccw
  arc A1 (-2496.523, 2783.5878) -> (-1776.8816, 2787.8567) centre (-2138.8294, 3144.3083) ccw
  arc A2 (-2496.523, 2783.5878) -> (-3632.2, 3251.2) centre (-3632.2, 1638.3) ccw
  line L3 (-3632.2, 3251.2) -> (-4241.8, 3251.2)
  line L4 (-4241.8, 3251.2) -> (-4241.8, 2438.4)
  line L5 (-4241.8, 2438.4) -> (-3710.305, 2438.4)
  arc A3 (-3710.305, 838.2) -> (-3710.305, 2438.4) centre (-3671.2525, 1638.3) ccw
  line L6 (-3710.305, 838.2) -> (-3730.625, 838.2)
  line L7 (-3730.625, 838.2) -> (-3730.625, 276.225)
  line L8 (-511.175, 250.825) -> (-511.175, 838.2)
  line L9 (-511.175, 838.2) -> (-482.6, 838.2)
  line L10 (-482.6, 838.2) -> (-482.6, 606.425)
  line L11 (-482.6, 606.425) -> (0, 606.425)
  line L12 (0, 606.425) -> (0, 838.2)
  line L13 (0, 838.2) -> (-531.495, 838.2)
  arc A4 (-531.495, 2438.4) -> (-531.495, 838.2) centre (-570.5475, 1638.3) ccw
  line L14 (-531.495, 2438.4) -> (0, 2438.4)
  line L15 (0, 2438.4) -> (0, 2670.175)
  line L16 (0, 2670.175) -> (-482.6, 2670.175)
  line L17 (-482.6, 2670.175) -> (-482.6, 2438.6051)
  line L18 (-482.6, 2438.6051) -> (-511.175, 2438.6051)
  line L19 (-511.175, 2438.6051) -> (-511.175, 3276.173)
  line L20 (-511.175, 3276.173) -> (-482.6, 3276.173)
  line L21 (-482.6, 3276.173) -> (-482.6, 3044.825)
  circle A5 centre (-3302, 2420.0312) radius 16
  circle A6 centre (-914.4, 845.0683) radius 16
  circle A7 centre (-863.6, 3192.4811) radius 16
  line L22 (-3730.6249, 3251.2) -> (-3730.6249, 2438.5075)
  line L23 (-3730.6249, 2438.5075) -> (-3759.1999, 2438.5075)
  line L24 (-3759.1999, 2438.5075) -> (-3759.1999, 3251.2)
  line L25 (-3759.1999, 3251.2) -> (-3730.6249, 3251.2)
  line L26 (0, 3025.775) -> (-609.6, 3025.775)
  arc A8 (-609.6, 3025.775) -> (-1598.1699, 2611.8586) centre (-609.6, 1638.3) ccw
  line L27 (0, 3044.825) -> (-609.6, 3044.825)
  arc A9 (-609.6, 3044.825) -> (-1611.7429, 2625.2256) centre (-609.6, 1638.3) ccw
  arc A10 (-2659.7206, 2619.009) -> (-1611.7429, 2625.2256) centre (-2138.8294, 3144.3083) ccw
  arc A11 (-2659.7206, 2619.009) -> (-3632.2, 3019.425) centre (-3632.2, 1638.3) ccw
  arc A12 (-2673.1342, 2605.482) -> (-1598.1699, 2611.8586) centre (-2138.8294, 3144.3083) ccw
  arc A13 (-2673.1342, 2605.482) -> (-3632.2, 3000.375) centre (-3632.2, 1638.3) ccw
  line L28 (-3632.2, 3019.425) -> (-4241.8, 3019.425)
  line L29 (-3632.2, 3000.375) -> (-4241.8, 3000.375)
  line L30 (-3730.625, 276.225) -> (-3632.2, 276.225)
  arc A14 (-3632.2, 276.225) -> (-2673.1342, 671.118) centre (-3632.2, 1638.3) ccw
  arc A15 (-1598.1699, 664.7414) -> (-2673.1342, 671.118) centre (-2138.8294, 132.2917) ccw
  arc A16 (-1598.1699, 664.7414) -> (-609.6, 250.825) centre (-609.6, 1638.3) ccw
  line L31 (-609.6, 250.825) -> (-511.175, 250.825)
  dimension "d112" = -250.825
  dimension "d113" = -231.775
  dimension "d114" = -231.775
  dimension "d115" = -250.825
  dimension "d116" = -231.775
  dimension "d117" = -250.825
extrude "Extrude18" add sketch "Sketch17" along normal blind 0.0279 contours L19 L22 L26 A8 L27 A9 A10 A11 A12 A13 L28 L29
sketch "Sketch18" plane through (0, 0, 50.8) normal (0, 0, 1) x (-1, 0, 0)
  line L0 (-3632.2, 3000.375) -> (-3730.6249, 3000.375)
  line L1 (-3730.6249, 3000.375) -> (-3730.6249, 2438.5075)
  line L2 (-3730.6249, 2438.5075) -> (-3759.1999, 2438.5075)
  line L3 (-3759.1999, 2438.5075) -> (-3759.1999, 3251.2)
  line L4 (-3759.1999, 3251.2) -> (-3730.6249, 3251.2)
  line L5 (-3730.6249, 3251.2) -> (-3730.6249, 3019.425)
  line L6 (-3730.6249, 3019.425) -> (-3632.2, 3019.425)
  arc A0 (-2659.7206, 2619.009) -> (-3632.2, 3019.425) centre (-3632.2, 1638.3) ccw
  arc A1 (-2659.7206, 2619.009) -> (-1611.7429, 2625.2256) centre (-2138.8294, 3144.3083) ccw
  arc A2 (-609.6, 3044.825) -> (-1611.7429, 2625.2256) centre (-609.6, 1638.3) ccw
  line L7 (-609.6, 3044.825) -> (-511.175, 3044.825)
  line L8 (-511.175, 3044.825) -> (-511.175, 3276.173)
  line L9 (-511.175, 3276.173) -> (-482.6, 3276.173)
  line L10 (-482.6, 3276.173) -> (-482.6, 3044.825)
  line L11 (-482.6, 3044.825) -> (0, 3044.825)
  line L12 (0, 3044.825) -> (0, 3276.6)
  line L13 (0, 3276.6) -> (-609.6, 3276.6)
  arc A3 (-609.6, 3276.6) -> (-1776.8816, 2787.8567) centre (-609.6, 1638.3) ccw
  arc A4 (-2496.523, 2783.5878) -> (-1776.8816, 2787.8567) centre (-2138.8294, 3144.3083) ccw
  arc A5 (-2496.523, 2783.5878) -> (-3632.2, 3251.2) centre (-3632.2, 1638.3) ccw
  line L14 (-3632.2, 3251.2) -> (-4241.8, 3251.2)
  line L15 (-4241.8, 3251.2) -> (-4241.8, 2438.4)
  line L16 (-4241.8, 2438.4) -> (-3710.305, 2438.4)
  arc A6 (-3710.305, 838.2) -> (-3710.305, 2438.4) centre (-3671.2525, 1638.3) ccw
  line L17 (-3710.305, 838.2) -> (-3730.625, 838.2)
  line L18 (-3730.625, 838.2) -> (-3730.625, 276.225)
  line L19 (-511.175, 250.825) -> (-511.175, 838.2)
  line L20 (-511.175, 838.2) -> (-482.6, 838.2)
  line L21 (-482.6, 838.2) -> (-482.6, 606.425)
  line L22 (-482.6, 606.425) -> (0, 606.425)
  line L23 (0, 606.425) -> (0, 838.2)
  line L24 (0, 838.2) -> (-531.495, 838.2)
  arc A7 (-531.495, 2438.4) -> (-531.495, 838.2) centre (-570.5475, 1638.3) ccw
  line L25 (-531.495, 2438.4) -> (0, 2438.4)
  line L26 (0, 2438.4) -> (0, 2670.175)
  line L27 (0, 2670.175) -> (-482.6, 2670.175)
  line L28 (-482.6, 2670.175) -> (-482.6, 2438.6051)
  line L29 (-482.6, 2438.6051) -> (-511.175, 2438.6051)
  line L30 (-511.175, 2438.6051) -> (-511.175, 3025.775)
  line L31 (-511.175, 3025.775) -> (-609.6, 3025.775)
  arc A8 (-609.6, 3025.775) -> (-1598.1699, 2611.8586) centre (-609.6, 1638.3) ccw
  arc A9 (-2673.1342, 2605.482) -> (-1598.1699, 2611.8586) centre (-2138.8294, 3144.3083) ccw
  arc A10 (-2673.1342, 2605.482) -> (-3632.2, 3000.375) centre (-3632.2, 1638.3) ccw
  circle A11 centre (-3302, 2420.0312) radius 16
  circle A12 centre (-914.4, 845.0683) radius 16
  circle A13 centre (-863.6, 3192.4811) radius 16
  line L32 (-511.175, 2689.225) -> (-609.6, 2689.225)
  arc A14 (-609.6, 2689.225) -> (-1358.3795, 2375.7094) centre (-609.6, 1638.3) ccw
  arc A15 (-2910.1061, 2366.5046) -> (-1358.3795, 2375.7094) centre (-2138.8294, 3144.3083) ccw
  arc A16 (-2910.1061, 2366.5046) -> (-3632.2, 2663.825) centre (-3632.2, 1638.3) ccw
  line L33 (-511.175, 2670.175) -> (-609.6, 2670.175)
  arc A17 (-609.6, 2670.175) -> (-1344.8064, 2362.3425) centre (-609.6, 1638.3) ccw
  arc A18 (-2923.5196, 2352.9776) -> (-1344.8064, 2362.3425) centre (-2138.8294, 3144.3083) ccw
  arc A19 (-2923.5196, 2352.9776) -> (-3632.2, 2644.775) centre (-3632.2, 1638.3) ccw
  line L34 (-4241.8, 2689.225) -> (-3716.0065, 2689.225)
  arc A20 (-3722.5331, 587.6732) -> (-3716.0065, 2689.225) centre (-3671.2525, 1638.3) ccw
  arc A21 (-3721.6044, 606.7006) -> (-3715.5992, 2670.175) centre (-3671.2525, 1638.3) ccw
  line L35 (-4241.8, 2670.175) -> (-3715.5992, 2670.175)
  line L36 (-3730.625, 276.225) -> (-3632.2, 276.225)
  arc A22 (-3632.2, 276.225) -> (-2673.1342, 671.118) centre (-3632.2, 1638.3) ccw
  arc A23 (-1598.1699, 664.7414) -> (-2673.1342, 671.118) centre (-2138.8294, 132.2917) ccw
  arc A24 (-1598.1699, 664.7414) -> (-609.6, 250.825) centre (-609.6, 1638.3) ccw
  line L37 (-609.6, 250.825) -> (-511.175, 250.825)
  dimension "d120" = -336.55
  dimension "d121" = 336.55
  dimension "d123" = -355.6
  dimension "d124" = 355.6
  dimension "d126" = 250.825
  dimension "d127" = -231.775
  constraint concentric A10 A19
  constraint concentric A10 A16
extrude "Extrude19" add sketch "Sketch18" along normal blind 0.0279 contours L1 A16 L34 A20 A21 L35 | A16 A18 A19 A20 A21 | L30 L32 A14 A15 A16 L33 A17 A18 A20